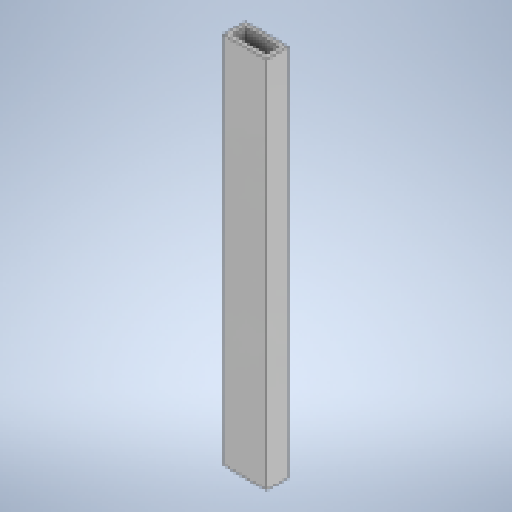
# Autodesk Inventor part: Beam
Saved by Autodesk Inventor 2023 (Build 270158000, 158)
## iProperties
Created: 2022-10-17
Part Number: Beam
Material: Aluminum 3004-O
Document SubType Name: Modeling
Designer: Miner
Density: 2.71043 g/cm^3
Appearance: Aluminum - Polished
Author: Miner
Autodesk Inventor part; units mm, degrees
ref_plane "YZ Plane" through (0, 0, 0) normal (1, 0, 0) x (0, 1, 0)
ref_plane "XZ Plane" through (0, 0, 0) normal (0, 1, 0) x (-1, 0, 0)
ref_plane "XY Plane" through (0, 0, 0) normal (0, 0, 1) x (1, 0, 0)
sketch "Sketch1" plane through (0, 0, 0) normal (0, 1, 0) x (-1, 0, 0)
  line L0 (0, 0) -> (-20.3, 0)
  line L1 (-20.3, 0) -> (-20.3, 10.3)
  line L2 (-20.3, 10.3) -> (0, 10.3)
  line L3 (0, 10.3) -> (0, 0)
  line L4 (-2.2, 2.2) -> (-18.1, 2.2)
  line L5 (-18.1, 2.2) -> (-18.1, 8.1)
  line L6 (-18.1, 8.1) -> (-2.2, 8.1)
  line L7 (-2.2, 8.1) -> (-2.2, 2.2)
  dimension "d0" = 20.3
  dimension "d1" = 10.3
  dimension "d2" = 2.2
  constraints: 16 end point, 4 parallel, 2 perpendicular, 1 horizontal, 3 other
  measures "d0" distance of L1.end L2.end
  measures "d1" distance of L0.end L1.end
  measures "d2" distance between parallel lines of L3 L7
extrude "Extrusion1" add sketch "Sketch1" along normal blind 150
extrude "Extrusion2" add sketch "Sketch1" against normal blind 25
body "Solid1"
